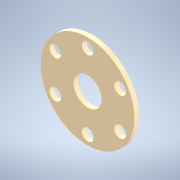
# Autodesk Inventor part: PTFESeal
Saved by Autodesk Inventor 2020 (Build 240168000, 168)
## iProperties
Created: 2019-09-29
Part Number: PTFESeal
Material: Polyethylene, High Density
Document SubType Name: Modeling
Designer: vmiguel
Density: 0.952 g/cm^3
Appearance: Smooth - Off-White
Author: vmiguel
Autodesk Inventor part; units mm, degrees
ref_plane "YZ Plane" through (0, 0, 0) normal (1, 0, 0) x (0, 1, 0)
ref_plane "XZ Plane" through (0, 0, 0) normal (0, 1, 0) x (-1, 0, 0)
ref_plane "XY Plane" through (0, 0, 0) normal (0, 0, 1) x (1, 0, 0)
sketch "Sketch1" plane through (0, 0, 0) normal (1, 0, 0) x (0, 1, 0)
  line L0 (0, 0) -> (0, -33.1818)
  line L1 (8, 2.1062) -> (20, 2.1062)
  line L2 (20, 2.1062) -> (20, 0.1062)
  line L3 (20, 0.1062) -> (8, 0.1062)
  line L4 (8, 0.1062) -> (8, 2.1062)
  dimension "d3" = 2
  dimension "d4" = 40
  dimension "d28" = 16
  constraints: 11 end point, 3 perpendicular, 1 horizontal, 1 vertical
  measures "d3" distance of L1.end L2.end
  measures "d4" diameter of L2 L0
  measures "d28" diameter of L4 L0
revolve "Revolution1" add sketch "Sketch1" angle 360 about axis through (0, 0, 0) along (0, 0, -1)
sketch "Sketch2" plane through (0, 0, 2.1062) normal (0, 0, 1) x (1, 0, 0)
  point P0 (0, 0)
  point P1 (0, 16)
  dimension "d6" = 16
  constraints: 1 vertical alignment
  measures "d6" distance of point (0, 16) point (0, 0)
hole "Hole1" at (0, 16, 2.1062) direction (0, 0, -1) diameter 5 end through all
pattern_circular "Circular Pattern1" count 6 over 360 about axis through (0, 0, 1.1062) along (0, 0, -1) of "Hole1"
body "Solid1"
